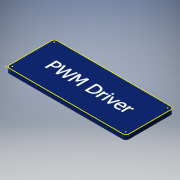
# Autodesk Inventor part: PWM Driver
Saved by Autodesk Inventor 2016 (Build 200138000, 138)
## iProperties
Created: 2015-10-05
Part Number: PWM Driver
Material: Generic
Document SubType Name: Modeling
Designer: powasar16
Density: 1 g/cm^3
Appearance: Default
Author: powasar16
Autodesk Inventor part; units mm, degrees
ref_plane "YZ Plane" through (0, 0, 0) normal (1, 0, 0) x (0, 1, 0)
ref_plane "XZ Plane" through (0, 0, 0) normal (0, 1, 0) x (-1, 0, 0)
ref_plane "XY Plane" through (0, 0, 0) normal (0, 0, 1) x (1, 0, 0)
sketch "Sketch1" plane through (0, 0, 0) normal (0, 1, 0) x (-1, 0, 0)
  line L0 (-1.5875, 0) -> (-61.9125, 0)
  line L1 (-63.5, -1.5875) -> (-63.5, -23.8125)
  line L2 (-61.9125, -25.4) -> (-1.5875, -25.4)
  line L3 (0, -23.8125) -> (0, -1.5875)
  arc A0 (0, -1.5875) -> (-1.5875, 0) centre (-1.5875, -1.5875) ccw
  line L4 (-31.75, -25.4) -> (-31.75, 0) construction
  line L5 (0, -12.7) -> (-63.5, -12.7) construction
  arc A1 (-61.9125, 0) -> (-63.5, -1.5875) centre (-61.9125, -1.5875) ccw
  arc A2 (-1.5875, -25.4) -> (0, -23.8125) centre (-1.5875, -23.8125) ccw
  arc A3 (-63.5, -23.8125) -> (-61.9125, -25.4) centre (-61.9125, -23.8125) ccw
  point P0 (0, 0)
  dimension "d2" = 3.175
  dimension "d5" = 60.325
  dimension "d6" = 60.325
  dimension "d7" = 22.225
  constraints: 12 end point, 9 symmetric about line, 8 point on circle, 4 centre point, 4 midpoint, 2 horizontal, 2 parallel, 2 tangent, 1 perpendicular, 1 vertical, 3 other
  measures "d2" diameter of A0
  measures "d5" distance of A3.centre A2.centre
  measures "d6" distance of A1.centre A0.centre
  measures "d7" distance of A3.centre A1.centre
extrude "Extrusion1" add sketch "Sketch1" along normal blind 2.54
sketch "Sketch2" plane through (0, 2.54, 0) normal (0, 1, 0) x (1, 0, 0)
  line L0 (61.9125, 25.4) -> (1.5875, 25.4) projected
  arc A0 (1.5875, 25.4) -> (0, 23.8125) centre (1.5875, 23.8125) ccw projected
  line L1 (0, 23.8125) -> (0, 1.5875) projected
  arc A1 (0, 1.5875) -> (1.5875, 0) centre (1.5875, 1.5875) ccw projected
  line L2 (1.5875, 0) -> (61.9125, 0) projected
  arc A2 (61.9125, 0) -> (63.5, 1.5875) centre (61.9125, 1.5875) ccw projected
  line L3 (63.5, 1.5875) -> (63.5, 23.8125) projected
  arc A3 (63.5, 23.8125) -> (61.9125, 25.4) centre (61.9125, 23.8125) ccw projected
  line L4 (9.9229, 16.0627) -> (63.8786, 16.0627) construction
  line L5 (63.8786, 16.0627) -> (63.8786, -1.5505) construction
  line L6 (63.8786, -1.5505) -> (9.9229, -1.5505) construction
  line L7 (9.9229, -1.5505) -> (9.9229, 16.0627) construction
  point P0 (0, 0)
  constraints: 2 other
body "Solid1"
